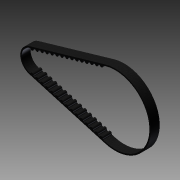
# Autodesk Inventor part: short turn belt
Saved by Autodesk Inventor 2012 (Build 160160000, 160)
## iProperties
Created: 2013-11-05
Part Number: short turn belt
Material: Default
Document SubType Name: Modeling
Designer: Bryce
Density: 1 g/cm^3
Author: Bryce
Autodesk Inventor part; units mm, degrees
ref_plane "YZ Plane" through (0, 0, 0) normal (1, 0, 0) x (0, 1, 0)
ref_plane "XZ Plane" through (0, 0, 0) normal (0, 1, 0) x (-1, 0, 0)
ref_plane "XY Plane" through (0, 0, 0) normal (0, 0, 1) x (1, 0, 0)
sketch "Sketch1" plane through (0, 0, 0) normal (0, 0, 1) x (1, 0, 0)
  arc A0 (-3.1756, 10.9007) -> (-3.1756, -10.9007) centre (0, 0) ccw
  arc A1 (72.9167, -33.0678) -> (72.9167, 33.0678) centre (82.55, 0) ccw
  line L0 (-3.1756, 10.9007) -> (72.9167, 33.0678)
  line L1 (-3.1756, -10.9007) -> (1.015, -12.1214)
  arc A2 (72.5402, -34.3603) -> (72.5402, 34.3603) centre (82.55, 0) ccw
  line L2 (72.5402, -34.3603) -> (-3.5521, -12.1931)
  arc A3 (-3.5521, 12.1931) -> (-3.5521, -12.1931) centre (0, 0) ccw
  line L3 (-3.5521, 12.1931) -> (72.5402, 34.3603)
  arc A4 (0.5844, -11.4345) -> (-2.4434, -10.5524) centre (-0.9808, -11.1697) ccw
  arc A5 (-3.1756, -10.9007) -> (-2.4434, -10.5524) centre (-3.0051, -10.3154) ccw
  arc A6 (0.5844, -11.4345) -> (1.015, -12.1214) centre (1.1855, -11.5362) ccw
  line L4 (1.015, -12.1214) -> (72.9167, -33.0678)
  line L5 (1.7992, -12.3499) -> (5.9898, -13.5707)
  arc A7 (5.5592, -12.8837) -> (2.5314, -12.0017) centre (3.994, -12.6189) ccw
  arc A8 (1.7992, -12.3499) -> (2.5314, -12.0017) centre (1.9697, -11.7646) ccw
  arc A9 (5.5592, -12.8837) -> (5.9898, -13.5707) centre (6.1603, -12.9854) ccw
  line L6 (6.774, -13.7992) -> (10.9646, -15.02)
  arc A10 (10.534, -14.333) -> (7.5062, -13.4509) centre (8.9688, -14.0682) ccw
  arc A11 (6.774, -13.7992) -> (7.5062, -13.4509) centre (6.9445, -13.2139) ccw
  arc A12 (10.534, -14.333) -> (10.9646, -15.02) centre (11.1351, -14.4347) ccw
  line L7 (11.7488, -15.2484) -> (15.9394, -16.4692)
  arc A13 (15.5088, -15.7822) -> (12.481, -14.9002) centre (13.9436, -15.5174) ccw
  arc A14 (11.7488, -15.2484) -> (12.481, -14.9002) centre (11.9193, -14.6632) ccw
  arc A15 (15.5088, -15.7822) -> (15.9394, -16.4692) centre (16.1099, -15.8839) ccw
  line L8 (16.7236, -16.6977) -> (20.9142, -17.9185)
  arc A16 (20.4836, -17.2315) -> (17.4558, -16.3494) centre (18.9184, -16.9667) ccw
  arc A17 (16.7236, -16.6977) -> (17.4558, -16.3494) centre (16.8941, -16.1124) ccw
  arc A18 (20.4836, -17.2315) -> (20.9142, -17.9185) centre (21.0847, -17.3332) ccw
  line L9 (21.6984, -18.1469) -> (25.889, -19.3677)
  arc A19 (25.4584, -18.6808) -> (22.4306, -17.7987) centre (23.8932, -18.4159) ccw
  arc A20 (21.6984, -18.1469) -> (22.4306, -17.7987) centre (21.8689, -17.5617) ccw
  arc A21 (25.4584, -18.6808) -> (25.889, -19.3677) centre (26.0595, -18.7824) ccw
  line L10 (26.6732, -19.5962) -> (30.8638, -20.817)
  arc A22 (30.4332, -20.13) -> (27.4054, -19.2479) centre (28.868, -19.8652) ccw
  arc A23 (26.6732, -19.5962) -> (27.4054, -19.2479) centre (26.8437, -19.0109) ccw
  arc A24 (30.4332, -20.13) -> (30.8638, -20.817) centre (31.0343, -20.2317) ccw
  line L11 (31.648, -21.0454) -> (35.8386, -22.2662)
  arc A25 (35.408, -21.5793) -> (32.3802, -20.6972) centre (33.8428, -21.3144) ccw
  arc A26 (31.648, -21.0454) -> (32.3802, -20.6972) centre (31.8185, -20.4602) ccw
  arc A27 (35.408, -21.5793) -> (35.8386, -22.2662) centre (36.0091, -21.681) ccw
  line L12 (36.6228, -22.4947) -> (40.8134, -23.7155)
  arc A28 (40.3828, -23.0285) -> (37.355, -22.1464) centre (38.8176, -22.7637) ccw
  arc A29 (36.6228, -22.4947) -> (37.355, -22.1464) centre (36.7933, -21.9094) ccw
  arc A30 (40.3828, -23.0285) -> (40.8134, -23.7155) centre (40.9839, -23.1302) ccw
  line L13 (41.5976, -23.9439) -> (45.7882, -25.1647)
  arc A31 (45.3576, -24.4778) -> (42.3298, -23.5957) centre (43.7924, -24.2129) ccw
  arc A32 (41.5976, -23.9439) -> (42.3298, -23.5957) centre (41.7681, -23.3587) ccw
  arc A33 (45.3576, -24.4778) -> (45.7882, -25.1647) centre (45.9587, -24.5795) ccw
  line L14 (46.5724, -25.3932) -> (50.763, -26.614)
  arc A34 (50.3324, -25.927) -> (47.3046, -25.045) centre (48.7672, -25.6622) ccw
  arc A35 (46.5724, -25.3932) -> (47.3046, -25.045) centre (46.7429, -24.8079) ccw
  arc A36 (50.3324, -25.927) -> (50.763, -26.614) centre (50.9335, -26.0287) ccw
  line L15 (51.5472, -26.8425) -> (55.7378, -28.0632)
  arc A37 (55.3072, -27.3763) -> (52.2794, -26.4942) centre (53.742, -27.1114) ccw
  arc A38 (51.5472, -26.8425) -> (52.2794, -26.4942) centre (51.7177, -26.2572) ccw
  arc A39 (55.3072, -27.3763) -> (55.7378, -28.0632) centre (55.9083, -27.478) ccw
  line L16 (56.522, -28.2917) -> (60.7126, -29.5125)
  arc A40 (60.282, -28.8255) -> (57.2542, -27.9435) centre (58.7168, -28.5607) ccw
  arc A41 (56.522, -28.2917) -> (57.2542, -27.9435) centre (56.6925, -27.7064) ccw
  arc A42 (60.282, -28.8255) -> (60.7126, -29.5125) centre (60.8831, -28.9272) ccw
  line L17 (61.4968, -29.741) -> (65.6874, -30.9617)
  arc A43 (65.2568, -30.2748) -> (62.229, -29.3927) centre (63.6916, -30.0099) ccw
  arc A44 (61.4968, -29.741) -> (62.229, -29.3927) centre (61.6673, -29.1557) ccw
  arc A45 (65.2568, -30.2748) -> (65.6874, -30.9617) centre (65.8579, -30.3765) ccw
  line L18 (66.4716, -31.1902) -> (70.6622, -32.411)
  arc A46 (70.2316, -31.724) -> (67.2038, -30.842) centre (68.6664, -31.4592) ccw
  arc A47 (66.4716, -31.1902) -> (67.2038, -30.842) centre (66.6421, -30.6049) ccw
  arc A48 (70.2316, -31.724) -> (70.6622, -32.411) centre (70.8327, -31.8257) ccw
  line L19 (0, 0) -> (82.55, 0) construction
  line L20 (-3.1756, 10.9007) -> (1.015, 12.1214)
  arc A49 (-2.4434, 10.5524) -> (0.5844, 11.4345) centre (-0.9808, 11.1697) ccw
  arc A50 (-2.4434, 10.5524) -> (-3.1756, 10.9007) centre (-3.0051, 10.3154) ccw
  arc A51 (1.015, 12.1214) -> (0.5844, 11.4345) centre (1.1855, 11.5362) ccw
  line L21 (1.7992, 12.3499) -> (5.9898, 13.5707)
  arc A52 (2.5314, 12.0017) -> (5.5592, 12.8837) centre (3.994, 12.6189) ccw
  arc A53 (2.5314, 12.0017) -> (1.7992, 12.3499) centre (1.9697, 11.7646) ccw
  arc A54 (5.9898, 13.5707) -> (5.5592, 12.8837) centre (6.1603, 12.9854) ccw
  line L22 (6.774, 13.7992) -> (10.9646, 15.02)
  arc A55 (7.5062, 13.4509) -> (10.534, 14.333) centre (8.9688, 14.0682) ccw
  arc A56 (7.5062, 13.4509) -> (6.774, 13.7992) centre (6.9445, 13.2139) ccw
  arc A57 (10.9646, 15.02) -> (10.534, 14.333) centre (11.1351, 14.4347) ccw
  line L23 (11.7488, 15.2484) -> (15.9394, 16.4692)
  arc A58 (12.481, 14.9002) -> (15.5088, 15.7822) centre (13.9436, 15.5174) ccw
  arc A59 (12.481, 14.9002) -> (11.7488, 15.2484) centre (11.9193, 14.6632) ccw
  arc A60 (15.9394, 16.4692) -> (15.5088, 15.7822) centre (16.1099, 15.8839) ccw
  line L24 (16.7236, 16.6977) -> (20.9142, 17.9185)
  arc A61 (17.4558, 16.3494) -> (20.4836, 17.2315) centre (18.9184, 16.9667) ccw
  arc A62 (17.4558, 16.3494) -> (16.7236, 16.6977) centre (16.8941, 16.1124) ccw
  arc A63 (20.9142, 17.9185) -> (20.4836, 17.2315) centre (21.0847, 17.3332) ccw
  line L25 (21.6984, 18.1469) -> (25.889, 19.3677)
  arc A64 (22.4306, 17.7987) -> (25.4584, 18.6808) centre (23.8932, 18.4159) ccw
  arc A65 (22.4306, 17.7987) -> (21.6984, 18.1469) centre (21.8689, 17.5617) ccw
  arc A66 (25.889, 19.3677) -> (25.4584, 18.6808) centre (26.0595, 18.7824) ccw
  line L26 (26.6732, 19.5962) -> (30.8638, 20.817)
  arc A67 (27.4054, 19.2479) -> (30.4332, 20.13) centre (28.868, 19.8652) ccw
  arc A68 (27.4054, 19.2479) -> (26.6732, 19.5962) centre (26.8437, 19.0109) ccw
  arc A69 (30.8638, 20.817) -> (30.4332, 20.13) centre (31.0343, 20.2317) ccw
  line L27 (31.648, 21.0454) -> (35.8386, 22.2662)
  arc A70 (32.3802, 20.6972) -> (35.408, 21.5793) centre (33.8428, 21.3144) ccw
  arc A71 (32.3802, 20.6972) -> (31.648, 21.0454) centre (31.8185, 20.4602) ccw
  arc A72 (35.8386, 22.2662) -> (35.408, 21.5793) centre (36.0091, 21.681) ccw
  line L28 (36.6228, 22.4947) -> (40.8134, 23.7155)
  arc A73 (37.355, 22.1464) -> (40.3828, 23.0285) centre (38.8176, 22.7637) ccw
  arc A74 (37.355, 22.1464) -> (36.6228, 22.4947) centre (36.7933, 21.9094) ccw
  arc A75 (40.8134, 23.7155) -> (40.3828, 23.0285) centre (40.9839, 23.1302) ccw
  line L29 (41.5976, 23.9439) -> (45.7882, 25.1647)
  arc A76 (42.3298, 23.5957) -> (45.3576, 24.4778) centre (43.7924, 24.2129) ccw
  arc A77 (42.3298, 23.5957) -> (41.5976, 23.9439) centre (41.7681, 23.3587) ccw
  arc A78 (45.7882, 25.1647) -> (45.3576, 24.4778) centre (45.9587, 24.5795) ccw
  line L30 (46.5724, 25.3932) -> (50.763, 26.614)
  arc A79 (47.3046, 25.045) -> (50.3324, 25.927) centre (48.7672, 25.6622) ccw
  arc A80 (47.3046, 25.045) -> (46.5724, 25.3932) centre (46.7429, 24.8079) ccw
  arc A81 (50.763, 26.614) -> (50.3324, 25.927) centre (50.9335, 26.0287) ccw
  line L31 (51.5472, 26.8425) -> (55.7378, 28.0632)
  arc A82 (52.2794, 26.4942) -> (55.3072, 27.3763) centre (53.742, 27.1114) ccw
  arc A83 (52.2794, 26.4942) -> (51.5472, 26.8425) centre (51.7177, 26.2572) ccw
  arc A84 (55.7378, 28.0632) -> (55.3072, 27.3763) centre (55.9083, 27.478) ccw
  line L32 (56.522, 28.2917) -> (60.7126, 29.5125)
  arc A85 (57.2542, 27.9435) -> (60.282, 28.8255) centre (58.7168, 28.5607) ccw
  arc A86 (57.2542, 27.9435) -> (56.522, 28.2917) centre (56.6925, 27.7064) ccw
  arc A87 (60.7126, 29.5125) -> (60.282, 28.8255) centre (60.8831, 28.9272) ccw
  line L33 (61.4968, 29.741) -> (65.6874, 30.9617)
  arc A88 (62.229, 29.3927) -> (65.2568, 30.2748) centre (63.6916, 30.0099) ccw
  arc A89 (62.229, 29.3927) -> (61.4968, 29.741) centre (61.6673, 29.1557) ccw
  arc A90 (65.6874, 30.9617) -> (65.2568, 30.2748) centre (65.8579, 30.3765) ccw
  line L34 (66.4716, 31.1902) -> (70.6622, 32.411)
  arc A91 (67.2038, 30.842) -> (70.2316, 31.724) centre (68.6664, 31.4592) ccw
  arc A92 (67.2038, 30.842) -> (66.4716, 31.1902) centre (66.6421, 30.6049) ccw
  arc A93 (70.6622, 32.411) -> (70.2316, 31.724) centre (70.8327, 31.8257) ccw
  line L35 (-3.0051, -10.3154) -> (1.1855, -11.5362) construction
  dimension "d0" = 82.55
  dimension "d1" = 11.3538
  dimension "d2" = 12.7
  dimension "d4" = 1.5875
  dimension "d5" = 0.6096
  dimension "d9" = 5.1816
  dimension "d16" = 34.4424
  dimension "d17" = 0.254
  constraints: 188 point on circle, 104 symmetric about line, 94 centre point, 72 end point, 15 tangent, 1 coincident, 1 equal radius, 1 horizontal alignment, 201 other
  measures "d0" distance of L19.end point (0, 0)
  measures "d1" radius of A0
  measures "d2" radius of A3
  measures "d4" radius of A4
  measures "d5" radius of A5
  measures "d9" distance of L1.start L5.start
  measures "d16" radius of A1
  measures "d17" distance from line of A4.centre L35
extrude "Extrusion1" add sketch "Sketch1" along normal blind 9 contours L0 A51 A49 A50 | A5 A4 A6 L1 | L0 A54 A52 A53 | A8 A7 A9 L4 | L0 A57 A55 A56 | A11 A10 A12 L4 | L0 A60 A58 A59 | A14 A13 A15 L4 | L0 A63 A61 A62 | A17 A16 A18 L4 | L0 A66 A64 A65 | A20 A19 A21 L4 | L0 A69 A67 A68 | A23 A22 A24 L4 | L0 A72 A70 A71 | A26 A25 A27 L4 | L0 A75 A73 A74 | A29 A28 A30 L4 | L0 A78 A76 A77 | A32 A31 A33 L4 | L0 A81 A79 A80 | A35 A34 A36 L4 | L0 A84 A82 A83 | A38 A37 A39 L4 | L0 A87 A85 A86 | A41 A40 A42 L4 | L0 A90 A88 A89 | A44 A43 A45 L4 | L0 A93 A91 A92 | A47 A46 A48 L4 | L2 A3 L3 A2
body "Solid1"
